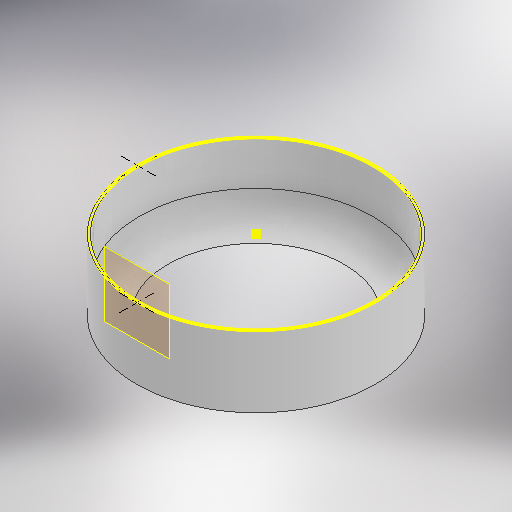
# Autodesk Inventor part: chevron_treads
Saved by Autodesk Inventor 2026 (Build 300175050, 175E)
## iProperties
Created: 2026-06-28
Part Number: chevron_treads
Material: Generic
Document SubType Name: Modeling
Designer: satom
Density: 1 g/cm^3
Appearance: Default
Author: satom
Autodesk Inventor part; units mm, degrees
ref_plane "YZ Plane" through (0, 0, 0) normal (1, 0, 0) x (0, 1, 0)
ref_plane "XZ Plane" through (0, 0, 0) normal (0, 1, 0) x (-1, 0, 0)
ref_plane "XY Plane" through (0, 0, 0) normal (0, 0, 1) x (1, 0, 0)
sketch "Sketch1" plane through (0, 0, 0) normal (0, 1, 0) x (-1, 0, 0)
  circle A0 centre (0, 0) radius 39.75
  circle A1 centre (0, 0) radius 40.5
  dimension "d0" = 79.5
  dimension "d1" = 81
  constraints: 2 centre point, 2 coincident
  measures "d0" diameter of A0
  measures "d1" diameter of A1
extrude "Extrusion1" add sketch "Sketch1" along normal blind 24
sketch "Sketch3" plane through (0, 24, 0) normal (0, 1, 0) x (1, 0, 0)
  circle A0 centre (0, 0) radius 40.5 projected
  circle A1 centre (0, 0) radius 39.75 projected
  point P0 (0, -40.5)
  point P1 (-39.75, 0)
  constraints: 1 horizontal alignment, 1 vertical alignment, 2 other
ref_plane "Work Plane2" through (0, 24, 40.5) normal (0, 0, 1) x (1, 0, 0)
sketch "Sketch7" plane through (0, 0, 0) normal (0, 0, 1) x (1, 0, 0)
  line L0 (39.75, 24) -> (39.75, 0) construction
  line L1 (0, 0) -> (-30, 0) construction
  line L2 (0, 0) -> (0, 12) construction
  line L3 (0, 12) -> (-39.75, 12) construction
  line L4 (0, 24) -> (-30, 24) construction
  ellipse E0 centre (0, 0.5748) end of major axis (-20.7169, 56.9851) minor radius 37.0729 (-40.2861, 24) -> (-40.231, 12) ccw projected
  line L5 (-30, 0) -> (-39.5989, 0)
  line L6 (-39.5989, 24) -> (-39.5989, 0)
  line L7 (-39.5989, 12) -> (-37.9524, 12) construction
  line L8 (-39.5989, 12) -> (-39.5989, 13.6344) construction
  arc A0 (-39.6019, 9.6019) -> (-30, 0) centre (-30, 9.6019) ccw
  line L9 (-30, 0) -> (-30, 9.6019) construction
  line L10 (-39.6019, 9.6019) -> (-30, 9.6019) construction
  line L11 (-30, 24) -> (-30, 13.1677) construction
  line L12 (-40.8323, 13.1677) -> (-30, 13.1677) construction
  line L13 (0, -7.1864) -> (0, 29.1977) projected
  point P0 (-39.5989, 9.3602)
  dimension "d24" = 30
  dimension "d25" = 12
  dimension "d26" = 39.75
  dimension "d27" = 30
  dimension "d28" = 90
  dimension "d29" = 90
  constraints: 24 end point, 3 horizontal, 2 point on circle, 2 point on line, 2 vertical, 1 centre point, 1 midpoint, 1 perpendicular, 1 tangent, 1 other
  measures "d24" distance of L1.start L1.end
  measures "d25" distance of L1.start L2.end
  measures "d26" distance of L2.end L3.end
  measures "d27" distance of L4.start L4.end
  measures "d28" angle of L10 L9
  measures "d29" angle of L11 L12
revolve "Revolution1" add sketch "Sketch7" angle 360 about axis through (0, -10, 0) along (0, 1, 0)
body "Solid1"
